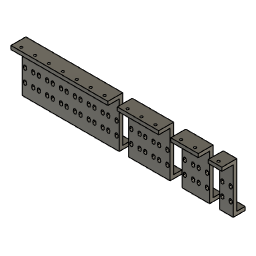
solenoid_holders_v2 (Autodesk Fusion 360 design; units mm, degrees)
Autodesk Fusion 360 part; units mm, degrees
sketch "Sketch1" plane through (0, 0, 0) normal (0, 0, 1) x (1, 0, 0)
  line L0 (0, 0) -> (23, 0)
  line L1 (23, 0) -> (23, 20)
  line L2 (23, 20) -> (0, 20)
  line L3 (0, 20) -> (0, 0)
  line L4 (0, 20) -> (23, 0) construction
  circle A0 centre (11.5, 10) radius 2.5
  line L5 (0, 0) -> (23, 0)
  line L6 (23, 0) -> (23, 6)
  line L7 (23, 6) -> (0, 6)
  line L8 (0, 6) -> (0, 0)
  dimension "d2" = 23
  dimension "d3" = 20
  dimension "d8" = 5
  dimension "d9" = 23
  dimension "d10" = 6
  constraint horizontal L0
  constraint vertical L1
  constraint horizontal L2
  constraint vertical L3
  constraint coincident L0.start L3.end
  constraint midpoint L4 A0.centre
  constraint horizontal L5
  constraint vertical L6
  constraint horizontal L7
  constraint vertical L8
  measures "d2" distance of L0.start L0.end
  measures "d3" distance of L0.start L2.end
  measures "d8" diameter of A0
  measures "d9" distance of L0.start L0.end
  measures "d10" distance of L0.start L7.end
extrude "Extrude1" add sketch "Sketch1" along normal blind 6 makes body 1
extrude "Extrude2" add sketch "Sketch1" along normal blind 83 contours L0 L1 L3 L5 L6 L7 L8 bodies 1
sketch "Sketch2" plane through (0, 6, 0) normal (0, 1, 0) x (-1, 0, 0)
  line L0 (-23, 6) -> (0, 6)
  line L1 (0, 6) -> (0, 83)
  line L2 (0, 83) -> (-23, 83)
  line L3 (-23, 83) -> (-23, 6)
  line L4 (-11.5, 83) -> (-11.5, 6) construction
  line L5 (-11.5, 6) -> (-11.5, 20) construction
  line L6 (-11.5, 20) -> (-18.5, 20) construction
  circle A0 centre (-18.5, 20) radius 2.5
  line L7 (-18.5, 20) -> (-18.5, 42) construction
  circle A1 centre (-18.5, 42) radius 2.5
  circle A2 centre (-4.5, 42) radius 2.5
  circle A3 centre (-4.5, 20) radius 2.5
  circle A4 centre (-18.5, 22.5) radius 2.5
  circle A5 centre (-18.5, 44.5) radius 2.5
  line L8 (-21, 42) -> (-21, 44.5)
  line L9 (-16, 44.5) -> (-16, 42)
  line L10 (-21, 20) -> (-21, 22.5)
  line L11 (-16, 22.5) -> (-16, 20)
  circle A6 centre (-4.5, 44.5) radius 2.5
  line L12 (-7, 44.5) -> (-7, 42)
  line L13 (-2, 42) -> (-2, 44.5)
  circle A7 centre (-4.5, 22.5) radius 2.5
  line L14 (-2, 20) -> (-2, 22.5)
  line L15 (-7, 22.5) -> (-7, 20)
  dimension "d19" = 14
  dimension "d20" = 7
  dimension "d21" = 5
  dimension "d22" = 22
  dimension "d23" = 5
  constraint midpoint L2 L4.start
  constraint midpoint L0 L4.end
  constraint perpendicular L0 L5
  constraint perpendicular L5 L6
  constraint coincident L6.end A0.centre
  constraint perpendicular L6 L7
  constraint coincident L7.end A1.centre
  constraint symmetric L4 A0 A3
  constraint symmetric L4 A1 A2
  constraint coincident A0 A4.centre
  constraint coincident L7 A4.centre
  constraint coincident L6.end A4
  constraint coincident A1 A5.centre
  constraint coincident L7.end A5
  constraint coincident A1 L8.start
  constraint coincident A5 L8.end
  constraint tangent A5 L8
  constraint parallel L7 L8
  constraint coincident A5 L9.start
  constraint coincident A1 L9.end
  constraint tangent A1 L9
  constraint parallel L7 L9
  constraint coincident A0 L10.start
  constraint coincident A4 L10.end
  constraint tangent A4 L10
  constraint parallel L7 L10
  constraint coincident A4 L11.start
  constraint coincident A0 L11.end
  constraint coincident L6 L11.end
  constraint tangent A0 L11
  constraint tangent A1 L8
  constraint symmetric L4 A4 A7
  constraint symmetric L4 A5 A6
  constraint symmetric L4 L8.start L13.start
  constraint symmetric L4 L8.end L13.end
  constraint symmetric L4 L9.start L12.start
  constraint symmetric L4 L9.end L12.end
  constraint symmetric L4 L10.start L14.start
  constraint symmetric L4 L10.end L14.end
  constraint symmetric L4 L11.start L15.start
  constraint symmetric L4 L11.end L15.end
  measures "d19" distance of L4.end L5.end
  measures "d20" distance of L5.end L6.end
  measures "d21" diameter of A0
  measures "d22" distance of L6.end L7.end
  measures "d23" diameter of A1
extrude "Extrude4" cut sketch "Sketch2" against normal up to surface (6 mm away) contours A0 A4 | A0 A4 L10 | A0 A4 L11 | A0 A4 | A0 A4 | A1 A5 | A1 A5 L8 | A1 A5 L9 | A1 A5 | A1 A5 | A2 A6 | A2 A6 L12 | A2 A6 L13 | A2 A6 | A2 A6 | A3 A7 | A3 A7 L15 | A3 A7 L14 | A3 A7 | A3 A7 bodies 1
sketch "Sketch9" plane through (0, 6, 0) normal (0, 1, 0) x (-1, 0, 0)
  arc A0 (-7, 42) -> (-2, 42) centre (-4.5, 42) ccw
  line L0 (-7, 42) -> (-7, 44.5)
  arc A1 (-2, 44.5) -> (-7, 44.5) centre (-4.5, 44.5) ccw
  line L1 (-2, 44.5) -> (-2, 42)
  arc A2 (-2, 22.5) -> (-7, 22.5) centre (-4.5, 22.5) ccw
  line L2 (-2, 22.5) -> (-2, 20)
  arc A3 (-7, 20) -> (-2, 20) centre (-4.5, 20) ccw
  line L3 (-7, 20) -> (-7, 22.5)
  line L4 (-21, 42) -> (-21, 44.5)
  arc A4 (-16, 44.5) -> (-21, 44.5) centre (-18.5, 44.5) ccw
  line L5 (-16, 44.5) -> (-16, 42)
  arc A5 (-21, 42) -> (-16, 42) centre (-18.5, 42) ccw
  line L6 (-21, 20) -> (-21, 22.5)
  arc A6 (-16, 22.5) -> (-21, 22.5) centre (-18.5, 22.5) ccw
  line L7 (-16, 22.5) -> (-16, 20)
  arc A7 (-21, 20) -> (-16, 20) centre (-18.5, 20) ccw
  line L8 (-23, 6) -> (0, 6)
  line L9 (0, 6) -> (0, 83)
  line L10 (0, 83) -> (-23, 83)
  line L11 (-23, 83) -> (-23, 6)
  line L12 (-23, 83) -> (0, 83)
  line L13 (0, 83) -> (0, 77)
  line L14 (0, 77) -> (-23, 77)
  line L15 (-23, 77) -> (-23, 83)
  dimension "d54" = 23
  dimension "d55" = 6
  constraint horizontal L12
  constraint vertical L13
  constraint horizontal L14
  constraint vertical L15
  constraint coincident L10.end L11.start
  measures "d54" distance of L10.end L9.end
  measures "d55" distance of L10.end L14.end
extrude "Extrude10" add sketch "Sketch9" against normal blind 25.25 contours L9 L10 L11 L12 L13 L14 L15 bodies 1
sketch "Sketch10" plane through (0, 0, 83) normal (0, 0, 1) x (-1, 0, 0)
  line L0 (0, -6) -> (0, 19.25)
  line L1 (0, 19.25) -> (-23, 19.25)
  line L2 (-23, 19.25) -> (-23, -6)
  line L3 (-23, -6) -> (0, -6)
  line L4 (0, 0) -> (-23, 0)
  line L5 (-11.5, 0) -> (-11.5, 13.25) construction
  circle A0 centre (-11.5, 13.25) radius 2
  dimension "d58" = 13.25
  dimension "d60" = 4
  constraint midpoint L4 L5.start
  constraint perpendicular L4 L5
  constraint coincident L5.end A0.centre
  measures "d58" distance of L5.start L5.end
  measures "d60" diameter of A0
extrude "Extrude11" cut sketch "Sketch10" against normal up to surface (6 mm away) contours A0 bodies 1
extrude "Extrude12" add 1 faces at (0, 4, 55.3333) along direction (-1, 0, 0) blind 3 on bodies 1 bodies 1
extrude "Extrude13" add 1 faces at (-3, 4, 55.3333) along direction (-1, 0, 0) blind 138 on bodies 1 bodies 1
sketch "Sketch11" plane through (0, 0, 6) normal (0, 0, 1) x (-1, 0, 0)
  line L0 (141, -6) -> (-23, -6)
  line L1 (-23, -6) -> (-23, -20)
  line L2 (-23, -20) -> (141, -20)
  line L3 (141, -20) -> (141, -6)
  circle A0 centre (-11.5, -10) radius 2.5
  line L4 (141, -20) -> (141, -10) construction
  line L5 (141, -10) -> (129.5, -10) construction
  circle A1 centre (129.5, -10) radius 2.5
  line L6 (129.5, -10) -> (106, -10) construction
  line L7 (106, -10) -> (82.5, -10) construction
  line L8 (82.5, -10) -> (59, -10) construction
  line L9 (59, -10) -> (35.5, -10) construction
  line L10 (35.5, -10) -> (12, -10) construction
  line L11 (12, -10) -> (-11.5, -10) construction
  circle A2 centre (106, -10) radius 2.5
  circle A3 centre (82.5, -10) radius 2.5
  circle A4 centre (59, -10) radius 2.5
  circle A5 centre (35.5, -10) radius 2.5
  circle A6 centre (12, -10) radius 2.5
  dimension "d68" = 10
  dimension "d69" = 11.5
  dimension "d70" = 5
  dimension "d71" = 23.5
  dimension "d72" = 23.5
  dimension "d73" = 23.5
  dimension "d74" = 23.5
  dimension "d75" = 23.5
  dimension "d76" = 23.5
  dimension "d77" = 5
  dimension "d78" = 5
  dimension "d79" = 5
  dimension "d80" = 5
  dimension "d81" = 5
  constraint coincident L2.end L3.start
  constraint perpendicular L2 L4
  constraint perpendicular L3 L5
  constraint coincident L5.end A1.centre
  constraint parallel L5 L6
  constraint parallel L6 L7
  constraint parallel L7 L8
  constraint parallel L8 L9
  constraint parallel L9 L10
  constraint parallel L10 L11
  constraint coincident L6.end L7.start
  constraint coincident L7.end L8.start
  constraint coincident L8.end L9.start
  constraint coincident L9.end L10.start
  constraint coincident L10.end L11.start
  measures "d68" distance of L2.end L4.end
  measures "d69" distance of L4.end L5.end
  measures "d70" diameter of A1
  measures "d71" distance of L5.end L6.end
  measures "d72" distance of L6.end L7.end
  measures "d73" distance of L7.end L8.end
  measures "d74" distance of L8.end L9.end
  measures "d75" distance of L9.end L10.end
  measures "d76" distance of L10.end A0.centre
  measures "d77" diameter of A2
  measures "d78" diameter of A3
  measures "d79" diameter of A4
  measures "d80" diameter of A5
  measures "d81" diameter of A6
extrude "Extrude14" cut sketch "Sketch11" against normal up to surface (6 mm away) contours A1 | A2 | A3 | A4 | A5 | A6 bodies 1
sketch "Sketch12" plane through (0, 6, 0) normal (0, 1, 0) x (-1, 0, 0)
  line L0 (-23, 83) -> (-23, 6)
  line L1 (-23, 6) -> (141, 6)
  line L2 (141, 6) -> (141, 83)
  line L3 (141, 83) -> (-23, 83)
  arc A0 (-7, 42) -> (-2, 42) centre (-4.5, 42) ccw
  line L4 (-7, 42) -> (-7, 44.5)
  arc A1 (-2, 44.5) -> (-7, 44.5) centre (-4.5, 44.5) ccw
  line L5 (-2, 44.5) -> (-2, 42)
  arc A2 (-2, 22.5) -> (-7, 22.5) centre (-4.5, 22.5) ccw
  line L6 (-2, 22.5) -> (-2, 20)
  arc A3 (-7, 20) -> (-2, 20) centre (-4.5, 20) ccw
  line L7 (-7, 20) -> (-7, 22.5)
  line L8 (-21, 42) -> (-21, 44.5)
  arc A4 (-16, 44.5) -> (-21, 44.5) centre (-18.5, 44.5) ccw
  line L9 (-16, 44.5) -> (-16, 42)
  arc A5 (-21, 42) -> (-16, 42) centre (-18.5, 42) ccw
  line L10 (-21, 20) -> (-21, 22.5)
  arc A6 (-16, 22.5) -> (-21, 22.5) centre (-18.5, 22.5) ccw
  line L11 (-16, 22.5) -> (-16, 20)
  arc A7 (-21, 20) -> (-16, 20) centre (-18.5, 20) ccw
  line L12 (-23, 83) -> (0.25, 83) construction
  line L13 (0.25, 83) -> (0.25, 6) construction
  arc A8 (16.5, 42) -> (21.5, 42) centre (19, 42) ccw
  arc A9 (21.5, 44.5) -> (16.5, 44.5) centre (19, 44.5) ccw
  line L14 (21.5, 42) -> (21.5, 44.5)
  line L15 (16.5, 44.5) -> (16.5, 42)
  line L16 (7.5, 42) -> (7.5, 44.5)
  arc A10 (7.5, 44.5) -> (2.5, 44.5) centre (5, 44.5) ccw
  line L17 (2.5, 44.5) -> (2.5, 42)
  arc A11 (2.5, 42) -> (7.5, 42) centre (5, 42) ccw
  arc A12 (7.5, 22.5) -> (2.5, 22.5) centre (5, 22.5) ccw
  line L18 (2.5, 22.5) -> (2.5, 20)
  arc A13 (2.5, 20) -> (7.5, 20) centre (5, 20) ccw
  line L19 (7.5, 20) -> (7.5, 22.5)
  arc A14 (16.5, 20) -> (21.5, 20) centre (19, 20) ccw
  line L20 (16.5, 22.5) -> (16.5, 20)
  arc A15 (21.5, 22.5) -> (16.5, 22.5) centre (19, 22.5) ccw
  line L21 (21.5, 20) -> (21.5, 22.5)
  line L22 (0.25, 83) -> (23.75, 83) construction
  line L23 (23.75, 83) -> (23.75, 6) construction
  line L24 (23.75, 83) -> (47.25, 83) construction
  line L25 (47.25, 83) -> (70.75, 83) construction
  line L26 (70.75, 83) -> (94.25, 83) construction
  line L27 (94.25, 83) -> (117.75, 83) construction
  line L28 (47.25, 83) -> (47.25, 6) construction
  line L29 (70.75, 83) -> (70.75, 6) construction
  line L30 (94.25, 83) -> (94.25, 6) construction
  line L31 (117.75, 83) -> (117.75, 6) construction
  line L32 (40, 42) -> (40, 44.5)
  arc A16 (45, 44.5) -> (40, 44.5) centre (42.5, 44.5) ccw
  line L33 (45, 44.5) -> (45, 42)
  arc A17 (40, 42) -> (45, 42) centre (42.5, 42) ccw
  line L34 (31, 44.5) -> (31, 42)
  arc A18 (31, 44.5) -> (26, 44.5) centre (28.5, 44.5) ccw
  line L35 (26, 42) -> (26, 44.5)
  arc A19 (26, 42) -> (31, 42) centre (28.5, 42) ccw
  arc A20 (31, 22.5) -> (26, 22.5) centre (28.5, 22.5) ccw
  line L36 (26, 20) -> (26, 22.5)
  arc A21 (26, 20) -> (31, 20) centre (28.5, 20) ccw
  line L37 (31, 22.5) -> (31, 20)
  arc A22 (45, 22.5) -> (40, 22.5) centre (42.5, 22.5) ccw
  line L38 (45, 22.5) -> (45, 20)
  arc A23 (40, 20) -> (45, 20) centre (42.5, 20) ccw
  line L39 (40, 20) -> (40, 22.5)
  line L40 (63.5, 44.5) -> (63.5, 42)
  arc A24 (68.5, 44.5) -> (63.5, 44.5) centre (66, 44.5) ccw
  line L41 (68.5, 42) -> (68.5, 44.5)
  arc A25 (63.5, 42) -> (68.5, 42) centre (66, 42) ccw
  line L42 (54.5, 42) -> (54.5, 44.5)
  arc A26 (54.5, 44.5) -> (49.5, 44.5) centre (52, 44.5) ccw
  line L43 (49.5, 44.5) -> (49.5, 42)
  arc A27 (49.5, 42) -> (54.5, 42) centre (52, 42) ccw
  arc A28 (68.5, 22.5) -> (63.5, 22.5) centre (66, 22.5) ccw
  line L44 (68.5, 20) -> (68.5, 22.5)
  arc A29 (63.5, 20) -> (68.5, 20) centre (66, 20) ccw
  line L45 (63.5, 22.5) -> (63.5, 20)
  line L46 (54.5, 20) -> (54.5, 22.5)
  arc A30 (54.5, 22.5) -> (49.5, 22.5) centre (52, 22.5) ccw
  line L47 (49.5, 22.5) -> (49.5, 20)
  arc A31 (49.5, 20) -> (54.5, 20) centre (52, 20) ccw
  arc A32 (92, 44.5) -> (87, 44.5) centre (89.5, 44.5) ccw
  line L48 (92, 44.5) -> (92, 42)
  line L49 (87, 42) -> (87, 44.5)
  arc A33 (87, 42) -> (92, 42) centre (89.5, 42) ccw
  arc A34 (78, 44.5) -> (73, 44.5) centre (75.5, 44.5) ccw
  line L50 (78, 44.5) -> (78, 42)
  line L51 (73, 42) -> (73, 44.5)
  arc A35 (73, 42) -> (78, 42) centre (75.5, 42) ccw
  arc A36 (92, 22.5) -> (87, 22.5) centre (89.5, 22.5) ccw
  line L52 (92, 22.5) -> (92, 20)
  arc A37 (87, 20) -> (92, 20) centre (89.5, 20) ccw
  line L53 (87, 20) -> (87, 22.5)
  arc A38 (78, 22.5) -> (73, 22.5) centre (75.5, 22.5) ccw
  line L54 (78, 22.5) -> (78, 20)
  arc A39 (73, 20) -> (78, 20) centre (75.5, 20) ccw
  line L55 (73, 20) -> (73, 22.5)
  line L56 (115.5, 42) -> (115.5, 44.5)
  arc A40 (115.5, 44.5) -> (110.5, 44.5) centre (113, 44.5) ccw
  line L57 (110.5, 44.5) -> (110.5, 42)
  arc A41 (110.5, 42) -> (115.5, 42) centre (113, 42) ccw
  line L58 (101.5, 42) -> (101.5, 44.5)
  arc A42 (101.5, 44.5) -> (96.5, 44.5) centre (99, 44.5) ccw
  line L59 (96.5, 44.5) -> (96.5, 42)
  arc A43 (96.5, 42) -> (101.5, 42) centre (99, 42) ccw
  arc A44 (101.5, 22.5) -> (96.5, 22.5) centre (99, 22.5) ccw
  line L60 (101.5, 20) -> (101.5, 22.5)
  arc A45 (96.5, 20) -> (101.5, 20) centre (99, 20) ccw
  line L61 (96.5, 22.5) -> (96.5, 20)
  line L62 (110.5, 22.5) -> (110.5, 20)
  arc A46 (115.5, 22.5) -> (110.5, 22.5) centre (113, 22.5) ccw
  line L63 (115.5, 20) -> (115.5, 22.5)
  arc A47 (110.5, 20) -> (115.5, 20) centre (113, 20) ccw
  line L64 (134, 42) -> (134, 44.5)
  arc A48 (139, 44.5) -> (134, 44.5) centre (136.5, 44.5) ccw
  line L65 (139, 44.5) -> (139, 42)
  arc A49 (134, 42) -> (139, 42) centre (136.5, 42) ccw
  line L66 (125, 44.5) -> (125, 42)
  arc A50 (125, 44.5) -> (120, 44.5) centre (122.5, 44.5) ccw
  line L67 (120, 42) -> (120, 44.5)
  arc A51 (120, 42) -> (125, 42) centre (122.5, 42) ccw
  arc A52 (125, 22.5) -> (120, 22.5) centre (122.5, 22.5) ccw
  line L68 (125, 22.5) -> (125, 20)
  arc A53 (120, 20) -> (125, 20) centre (122.5, 20) ccw
  line L69 (120, 20) -> (120, 22.5)
  line L70 (134, 20) -> (134, 22.5)
  arc A54 (139, 22.5) -> (134, 22.5) centre (136.5, 22.5) ccw
  line L71 (139, 22.5) -> (139, 20)
  arc A55 (134, 20) -> (139, 20) centre (136.5, 20) ccw
  dimension "d84" = 23.25
  dimension "d85" = 23.5
  dimension "d86" = 23.5
  dimension "d87" = 23.5
  dimension "d88" = 23.5
  dimension "d89" = 23.5
  constraint coincident L0.start L3.end
  constraint perpendicular L0 L12
  constraint coincident L1 L13.end
  constraint perpendicular L1 L13
  constraint symmetric A0.start L13 L16.start
  constraint symmetric A0.end L13 L17.end
  constraint symmetric A0 L13 A11
  constraint symmetric L4.end L13 L16.end
  constraint symmetric A1.start L13 A10.end
  constraint symmetric A1 L13 A10
  constraint symmetric A2.start L13 A12.end
  constraint symmetric A2.end L13 A12.start
  constraint symmetric A2 L13 A12
  constraint symmetric L6.end L13 L18.end
  constraint symmetric A3.start L13 A13.end
  constraint symmetric A3 L13 A13
  constraint symmetric L8.start L13 A8.end
  constraint symmetric L8.end L13 A9.start
  constraint symmetric A4.start L13 A9.end
  constraint symmetric A4 L13 A9
  constraint symmetric L9.end L13 A8.start
  constraint symmetric A5 L13 A8
  constraint symmetric L10.start L13 A14.end
  constraint symmetric L10.end L13 A15.start
  constraint symmetric A6.start L13 L20.start
  constraint symmetric A6 L13 A15
  constraint symmetric L11.end L13 A14.start
  constraint symmetric A7 L13 A14
  constraint perpendicular L13 L22
  constraint coincident L1 L23.end
  constraint perpendicular L1 L23
  constraint perpendicular L23 L24
  constraint parallel L3 L25
  constraint parallel L3 L26
  constraint parallel L3 L27
  constraint coincident L1 L28.end
  constraint perpendicular L1 L28
  constraint coincident L1 L29.end
  constraint perpendicular L1 L29
  constraint perpendicular L27 L30
  constraint coincident L1 L31.end
  constraint perpendicular L1 L31
  constraint symmetric A8.end L23 L35.start
  constraint symmetric A8.start L23 L34.end
  constraint symmetric A8 L23 A19
  constraint symmetric A9.end L23 L34.start
  constraint symmetric A9.start L23 A18.end
  constraint symmetric A9 L23 A18
  constraint symmetric L16.start L23 L32.start
  constraint symmetric L16.end L23 L32.end
  constraint symmetric A10.end L23 A16.start
  constraint symmetric A10 L23 A16
  constraint symmetric L17.end L23 L33.end
  constraint symmetric A11 L23 A17
  constraint symmetric A12.end L23 A22.start
  constraint symmetric A12.start L23 A22.end
  constraint symmetric A12 L23 A22
  constraint symmetric L18.end L23 L38.end
  constraint symmetric A13.end L23 A23.start
  constraint symmetric A13 L23 A23
  constraint symmetric A14.end L23 L36.start
  constraint symmetric A14.start L23 A21.end
  constraint symmetric A14 L23 A21
  constraint symmetric L20.start L23 A20.start
  constraint symmetric A15.start L23 A20.end
  constraint symmetric A15 L23 A20
  constraint symmetric L28 L32.start L42.start
  constraint symmetric L28 L32.end L42.end
  constraint symmetric L28 A16.start A26.end
  constraint symmetric L28 A16 A26
  constraint symmetric L28 L33.end L43.end
  constraint symmetric L28 A17 A27
  constraint symmetric L28 L34.start L40.start
  constraint symmetric L28 L34.end L40.end
  constraint symmetric L28 A18.end A24.start
  constraint symmetric L28 A18 A24
  constraint symmetric L28 L35.start L41.start
  constraint symmetric L28 A19 A25
  constraint symmetric L28 A20.end A28.start
  constraint symmetric L28 A20.start A28.end
  constraint symmetric L28 A20 A28
  constraint symmetric L28 L36.start L44.start
  constraint symmetric L28 A21.end A29.start
  constraint symmetric L28 A21 A29
  constraint symmetric L28 A22.end L46.end
  constraint symmetric L28 A22.start A30.end
  constraint symmetric L28 A22 A30
  constraint symmetric L28 L38.end L47.end
  constraint symmetric L28 A23.start L46.start
  constraint symmetric L28 A23 A31
  constraint symmetric L29 L40.start A34.start
  constraint symmetric L29 L40.end L50.end
  constraint symmetric L29 A24.start A34.end
  constraint symmetric L29 A24 A34
  constraint symmetric L29 L41.start L51.start
  constraint symmetric L29 A25 A35
  constraint symmetric L29 L42.start L49.start
  constraint symmetric L29 L42.end A32.end
  constraint symmetric L29 A26.end A32.start
  constraint symmetric L29 A26 A32
  constraint symmetric L29 L43.end L48.end
  constraint symmetric L29 A27 A33
  constraint symmetric L29 A28.end A38.start
  constraint symmetric L29 A28.start A38.end
  constraint symmetric L29 A28 A38
  constraint symmetric L29 L44.start A39.start
  constraint symmetric L29 A29.start L54.end
  constraint symmetric L29 A29 A39
  constraint symmetric L29 L46.start A37.start
  constraint symmetric L29 L46.end A36.end
  constraint symmetric L29 A30.end A36.start
  constraint symmetric L29 A30 A36
  constraint symmetric L29 L47.end L52.end
  constraint symmetric L29 A31 A37
  constraint symmetric L30 A32.end L58.end
  constraint symmetric L30 A32.start A42.end
  constraint symmetric L30 A32 A42
  constraint symmetric L30 L48.end L59.end
  constraint symmetric L30 L49.start L58.start
  constraint symmetric L30 A33 A43
  constraint symmetric L30 A34.end L56.end
  constraint symmetric L30 A34.start A40.end
  constraint symmetric L30 A34 A40
  constraint symmetric L30 L50.end L57.end
  constraint symmetric L30 L51.start L56.start
  constraint symmetric L30 A35 A41
  constraint symmetric L30 A36.end A44.start
  constraint symmetric L30 A36.start A44.end
  constraint symmetric L30 A36 A44
  constraint symmetric L30 L52.end A45.start
  constraint symmetric L30 A37.start L60.start
  constraint symmetric L30 A37 A45
  constraint symmetric L30 A38.end A46.start
  constraint symmetric L30 A38.start L62.start
  constraint symmetric L30 A38 A46
  constraint symmetric L30 L54.end L62.end
  constraint symmetric L30 A39.start L63.start
  constraint symmetric L30 A39 A47
  constraint symmetric L31 L56.start L67.start
  constraint symmetric L31 L56.end A50.end
  constraint symmetric L31 A40.end L66.start
  constraint symmetric L31 A40 A50
  constraint symmetric L31 L57.end L66.end
  constraint symmetric L31 A41 A51
  constraint symmetric L31 L58.start L64.start
  constraint symmetric L31 L58.end L64.end
  constraint symmetric L31 A42.end A48.start
  constraint symmetric L31 A42 A48
  constraint symmetric L31 L59.end L65.end
  constraint symmetric L31 A43 A49
  constraint symmetric L31 A44.end A54.start
  constraint symmetric L31 A44.start L70.end
  constraint symmetric L31 A44 A54
  constraint symmetric L31 L60.start L70.start
  constraint symmetric L31 A45.start L71.end
  constraint symmetric L31 A45 A55
  constraint symmetric L31 L62.start A52.start
  constraint symmetric L31 L62.end L68.end
  constraint symmetric L31 A46.start A52.end
  constraint symmetric L31 A46 A52
  constraint symmetric L31 L63.start A53.start
  constraint symmetric L31 A47 A53
  measures "d84" distance of L0.start L12.end
  measures "d85" distance of L12.end L22.end
  measures "d86" distance of L22.end L24.end
  measures "d87" distance of L24.end L25.end
  measures "d88" distance of L25.end L26.end
  measures "d89" distance of L26.end L27.end
extrude "Extrude15" cut sketch "Sketch12" against normal up to surface (6 mm away) contours A8 A9 L14 L15 | L16 A10 L17 A11 | A12 L18 A13 L19 | A14 L20 A15 L21 | L32 A16 L33 A17 | L34 A18 L35 A19 | A20 L36 A21 L37 | A22 L38 A23 L39 | L40 A24 L41 A25 | L42 A26 L43 A27 | A28 L44 A29 L45 | L46 A30 L47 A31 | A32 L48 L49 A33 | A34 L50 L51 A35 | A36 L52 A37 L53 | A38 L54 A39 L55 | L56 A40 L57 A41 | L58 A42 L59 A43 | A44 L60 A45 L61 | L62 A46 L63 A47 | L64 A48 L65 A49 | L66 A50 L67 A51 | A52 L68 A53 L69 | L70 A54 L71 A55 bodies 1
sketch "Sketch13" plane through (0, 0, 83) normal (0, 0, 1) x (-1, 0, 0)
  circle A0 centre (-11.5, 13.25) radius 2
  line L0 (141, 19.25) -> (-23, 19.25)
  line L1 (-23, 19.25) -> (-23, -6)
  line L2 (-23, -6) -> (141, -6)
  line L3 (141, -6) -> (141, 19.25)
  line L4 (-11.5, 13.25) -> (12, 13.25) construction
  line L5 (12, 13.25) -> (35.5, 13.25) construction
  line L6 (35.5, 13.25) -> (59, 13.25) construction
  line L7 (59, 13.25) -> (82.5, 13.25) construction
  line L8 (82.5, 13.25) -> (106, 13.25) construction
  line L9 (106, 13.25) -> (129.5, 13.25) construction
  circle A1 centre (12, 13.25) radius 2
  circle A2 centre (35.5, 13.25) radius 2
  circle A3 centre (59, 13.25) radius 2
  circle A4 centre (82.5, 13.25) radius 2
  circle A5 centre (106, 13.25) radius 2
  circle A6 centre (129.5, 13.25) radius 2
  dimension "d92" = 23.5
  dimension "d93" = 23.5
  dimension "d94" = 23.5
  dimension "d95" = 23.5
  dimension "d96" = 23.5
  dimension "d97" = 23.5
  dimension "d98" = 4
  dimension "d99" = 4
  dimension "d100" = 4
  dimension "d101" = 4
  dimension "d102" = 4
  dimension "d103" = 4
  constraint coincident A0.centre L4.start
  constraint parallel L0 L4
  constraint parallel L4 L5
  constraint parallel L5 L6
  constraint parallel L6 L7
  constraint parallel L7 L8
  constraint parallel L8 L9
  constraint coincident L4.end L5.start
  constraint coincident L5.end L6.start
  constraint coincident L6.end L7.start
  constraint coincident L7.end L8.start
  constraint coincident L8.end L9.start
  constraint coincident L9.end A6.centre
  measures "d92" distance of A0.centre L4.end
  measures "d93" distance of L4.end L5.end
  measures "d94" distance of L5.end L6.end
  measures "d95" distance of L6.end L7.end
  measures "d96" distance of L7.end L8.end
  measures "d97" distance of L8.end L9.end
  measures "d98" diameter of A1
  measures "d99" diameter of A2
  measures "d100" diameter of A3
  measures "d101" diameter of A4
  measures "d102" diameter of A5
  measures "d103" diameter of A6
extrude "Extrude16" cut sketch "Sketch13" against normal up to surface (6 mm away) contours A1 | A2 | A3 | A4 | A5 | A6 bodies 1
copy_body "CopyPasteBodies1" bodies 1 makes body 2
move_body "Move1" bodies 2 to x (1, 0, 0) y (0, 1, 0) z (0, 0, 1) at (180, 0, 0)
copy_body "Body->Comp1" bodies 1 removing the originals makes body 3 in component "white_key_octave"
ref_plane "WorkPlane1" through (109.25, 0.375, 41.5) normal (-1, 0, 0) x (0, 0, 1)
split "Split1" by plane through (109.25, 0.375, 41.5) normal (-1, 0, 0) bodies 2 makes body 4 at (76.2312, 6, 70.9791)
ref_plane "WorkPlane2" through (156.25, 0.375, 41.5) normal (-1, 0, 0) x (0, 0, 1)
split "Split2" by plane through (156.25, 0.375, 41.5) normal (-1, 0, 0) bodies 2 makes body 5 at (131.3521, 0, 66.9791)
delete_body "RemoveBody2" bodies 2
move_body "Move2" bodies 5 to x (1, 0, 0) y (0, 1, 0) z (0, 0, 1) at (20, 0, 0)
copy_body "Body->Comp2" bodies 4 removing the originals makes body 6 in component "black_key_3"
copy_body "CopyPasteBodies2" bodies 5 makes body 7
move_body "Move3" bodies 7 to x (1, 0, 0) y (0, 1, 0) z (0, 0, 1) at (70, 0, 0)
copy_body "Body->Comp4" bodies 5 removing the originals makes body 8 in component "black_key_2 (1)"
ref_plane "WorkPlane3" through (223, 0.375, 41.5) normal (1, 0, 0) x (0, 0, -1)
split "Split3" by plane through (223, 0.375, 41.5) normal (1, 0, 0) bodies 7 makes body 9 at (236.6122, 6, 70.9424)
delete_body "RemoveBody6" bodies 7
move_body "Move4" bodies 9 to x (1, 0, 0) y (0, 1, 0) z (0, 0, 1) at (-30, 0, 0)
copy_body "Body->Comp5" bodies 9 removing the originals makes body 10 in component "single_key"
extrude "Extrude1'" cut 1 faces at (109.25, 4, 55.3333) along direction (-1, 0, 0) blind 0.25 on bodies 6 bodies 6 in component "black_key_3"
extrude "Extrude1''" cut 1 faces at (176.25, 4, 55.3333) along direction (-1, 0, 0) blind 0.25 on bodies 8 bodies 8 in component "black_key_2 (1)"
extrude "Extrude2'" cut 1 faces at (129.25, 4, 55.3333) along direction (1, 0, 0) blind 0.25 on bodies 8 bodies 8 in component "black_key_2 (1)"
extrude "Extrude1'''" cut 1 faces at (216.25, 4, 55.3333) along direction (-1, 0, 0) blind 0.25 on bodies 10 bodies 10 in component "single_key"
component "white_key_octave" placed x (1, 0, 0) y (0, 1, 0) z (0, 0, 1) at (0, 0, 0)
component "black_key_3" placed x (1, 0, 0) y (0, 1, 0) z (0, 0, 1) at (0, 0, 0)
component "black_key_2 (1)" placed x (1, 0, 0) y (0, 1, 0) z (0, 0, 1) at (0, 0, 0)
component "single_key" placed x (1, 0, 0) y (0, 1, 0) z (0, 0, 1) at (0, 0, 0)
equation "mount_width = 23 mm"
equation "d2 = mount_width"
equation "d3 = extrusion_width"
equation "extrusion_width = 20 mm"
equation "bolt_hole_diameter = 5 mm"
equation "solenoid_depth = 26.5 mm"
equation "mount_thickness = 6 mm"
equation "d8 = bolt_hole_diameter"
equation "d9 = mount_width"
equation "d10 = mount_thickness"
equation "d11 = mount_thickness"
equation "d13 = mount_thickness + solenoid_mount_height"
equation "solenoid_mounting_hole_y_spacing = 22 mm"
equation "solenoid_mounting_hole_x_spacing = 14 mm"
equation "solenoid_mounting_hole_bottom_offset = 14 mm"
equation "solenoid_mount_height = 77 mm"
equation "d19 = solenoid_mounting_hole_bottom_offset"
equation "d20 = solenoid_mounting_hole_x_spacing / 2"
equation "d21 = bolt_hole_diameter"
equation "d22 = solenoid_mounting_hole_y_spacing"
equation "d23 = bolt_hole_diameter"
equation "m4_nut_recess_radius = 3.5 mm"
equation "m4_recess_top_offset = 8 mm"
equation "nut_recess_depth = 3.25 mm"
equation "d54 = mount_width"
equation "d55 = mount_thickness"
equation "d56 = -1 * ( mount_thickness * 2 + solenoid_depth / 2 )"
equation "d58 = solenoid_depth / 2"
equation "tight_m4_bolt_hole = 4 mm"
equation "d60 = tight_m4_bolt_hole"
equation "thickness_between_solenoids = 0.5 mm"
equation "d64 = thickness_between_solenoids * 6"
equation "d66 = mount_width * 6"
equation "d68 = extrusion_width / 2"
equation "d69 = mount_width / 2"
equation "d70 = bolt_hole_diameter"
equation "d71 = mount_width + thickness_between_solenoids"
equation "d72 = mount_width + thickness_between_solenoids"
equation "d73 = mount_width + thickness_between_solenoids"
equation "d74 = mount_width + thickness_between_solenoids"
equation "d75 = mount_width + thickness_between_solenoids"
equation "d76 = mount_width + thickness_between_solenoids"
equation "d77 = bolt_hole_diameter"
equation "d78 = bolt_hole_diameter"
equation "d79 = bolt_hole_diameter"
equation "d80 = bolt_hole_diameter"
equation "d81 = bolt_hole_diameter"
equation "d84 = mount_width + thickness_between_solenoids / 2"
equation "d85 = mount_width + thickness_between_solenoids"
equation "d86 = mount_width + thickness_between_solenoids"
equation "d87 = mount_width + thickness_between_solenoids"
equation "d88 = mount_width + thickness_between_solenoids"
equation "d89 = mount_width + thickness_between_solenoids"
equation "d92 = mount_width + thickness_between_solenoids"
equation "d93 = mount_width + thickness_between_solenoids"
equation "d94 = mount_width + thickness_between_solenoids"
equation "d95 = mount_width + thickness_between_solenoids"
equation "d96 = mount_width + thickness_between_solenoids"
equation "d97 = mount_width + thickness_between_solenoids"
equation "d98 = tight_m4_bolt_hole"
equation "d99 = tight_m4_bolt_hole"
equation "d100 = tight_m4_bolt_hole"
equation "d101 = tight_m4_bolt_hole"
equation "d102 = tight_m4_bolt_hole"
equation "d103 = tight_m4_bolt_hole"
equation "d106 = -1 * ( mount_width + thickness_between_solenoids / 2 + 2 * ( mount_width + thickness_between_solenoids ) )"
equation "d107 = -2 * ( mount_width + thickness_between_solenoids )"
equation "d108 = -1 * ( mount_width + thickness_between_solenoids / 2 )"
equation "d109 = -( thickness_between_solenoids / 2 )"
equation "d111 = -( thickness_between_solenoids / 2 )"
equation "d113 = -( thickness_between_solenoids / 2 )"
equation "d115 = -( thickness_between_solenoids / 2 )"
